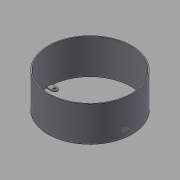
# Autodesk Inventor part: frame5
Saved by Autodesk Inventor 2015 (Build 190159000, 159)
## iProperties
Created: 2016-10-20
Part Number: frame5
Material: Generic
Document SubType Name: Modeling
Designer: Paulo Loma
Density: 1 g/cm^3
Appearance: Default
Author: Paulo Loma
Autodesk Inventor part; units mm, degrees
ref_plane "YZ Plane" through (0, 0, 0) normal (1, 0, 0) x (0, 1, 0)
ref_plane "XZ Plane" through (0, 0, 0) normal (0, 1, 0) x (-1, 0, 0)
ref_plane "XY Plane" through (0, 0, 0) normal (0, 0, 1) x (1, 0, 0)
sketch "Sketch1" plane through (0, 0, 0) normal (0, 0, 1) x (1, 0, 0)
  circle A0 centre (0, 0) radius 46.8237
  circle A1 centre (-39.5, 0) radius 1.5
  arc A2 (-39.5, -3) -> (-39.5, 3) centre (-39.5, 0) ccw
  line L0 (-39.5, -3) -> (-45.7254, -3)
  line L1 (-39.5, 3) -> (-45.7254, 3)
  circle A3 centre (39.5, 0) radius 1.5
  arc A4 (39.5, 3) -> (39.5, -3) centre (39.5, 0) ccw
  line L2 (39.5, 3) -> (45.7254, 3)
  line L3 (39.5, -3) -> (45.7254, -3)
  arc A5 (-45.7254, -3) -> (45.7254, -3) centre (0, 0) ccw
  arc A6 (45.7254, 3) -> (-45.7254, 3) centre (0, 0) ccw
  point P0 (0, 0)
  constraints: 8 end point, 8 point on circle, 7 centre point, 2 coincident, 2 horizontal, 1 parallel, 1 tangent
extrude "Extrusion1" add sketch "Sketch1" along normal blind 1
sketch "Sketch2" plane through (0, 0, 1) normal (0, 0, 1) x (1, 0, 0)
  circle A0 centre (0, 0) radius 46.8237 projected
  circle A1 centre (0, 0) radius 45.8237
  point P0 (0, 0)
  dimension "d5" = 1
  constraints: 1 centre point
  measures "d5" radial gap between concentric circles of A0 A1
extrude "Extrusion2" add sketch "Sketch2" along normal blind 38
body "Solid1"
